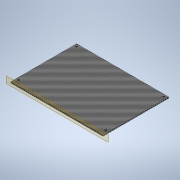
# Autodesk Inventor part: s_carbon_plate1
Saved by Autodesk Inventor 2022 (Build 260153000, 153)
## iProperties
Created: 2021-08-20
Part Number: s_carbon_plate1
Material: CFRP
Document SubType Name: Sheet Metal
Designer: yuta0
Density: 1.43 g/cm^3
Sheet Metal Rule: Default_mm
Appearance: カーボンファイバー
Mass: 103.386 g
Surface Area: 742.83 cm^2
Volume: 72.2979 cm^3
Author: yuta0
Autodesk Inventor part; units mm, degrees
ref_plane "YZ Plane" through (0, 0, 0) normal (1, 0, 0) x (0, 1, 0)
ref_plane "XZ Plane" through (0, 0, 0) normal (0, 1, 0) x (-1, 0, 0)
ref_plane "XY Plane" through (0, 0, 0) normal (0, 0, 1) x (1, 0, 0)
sketch "スケッチ1" plane through (0, 0, 0) normal (0, 1, 0) x (-1, 0, 0)
  line L0 (-87.5, 105) -> (87.5, 105)
  line L1 (87.5, 105) -> (87.5, -105)
  line L2 (87.5, -105) -> (-87.5, -105)
  line L3 (-87.5, -105) -> (-87.5, 105)
  line L4 (-87.5, 105) -> (87.5, -105) construction
  line L5 (87.5, 105) -> (-87.5, -105) construction
  point P0 (0, 0)
  dimension "d0" = 210
  dimension "d1" = 175
  measures "d0" distance of L0.end L1.end
  measures "d1" distance of L0.start L0.end
extrude "プレート1" add sketch "スケッチ1" along normal blind 2
sketch "スケッチ5" plane through (0, 2, 0) normal (0, 1, 0) x (1, 0, 0)
  line L0 (-24, -101) -> (34.6, -101)
  line L1 (34.6, -101) -> (34.6, -67)
  line L2 (34.6, -67) -> (-24, -67)
  line L3 (-24, -67) -> (-24, -101)
  line L4 (-24, -101) -> (34.6, -67) construction
  line L5 (34.6, -101) -> (-24, -67) construction
  line L6 (87.5, -105) -> (-87.5, -105) projected
  point P0 (0, 0)
  point P1 (0, -84)
  point P2 (5.3, -84)
  point P3 (5.3, -84)
  dimension "d31" = 58.6
  dimension "d32" = 24
  dimension "d33" = 34
  dimension "d78" = 4
  constraints: 12 end point, 3 midpoint, 2 parallel, 1 horizontal, 1 horizontal alignment, 1 perpendicular, 1 vertical alignment
  measures "d31" distance of L1.end L2.end
  measures "d32" distance from line of L3 point (0, -84)
  measures "d33" distance of L0.end L1.end
  measures "d78" distance between parallel lines of L6 L0
hole "穴3" at (34.6, 2, 67) at (34.6, 2, 101) at (-24, 2, 67) at (-24, 2, 101) direction (0, -1, 0) diameter 4.3 end through all clearance for "Socket Head Cap Screw" size "M4" standard "Ansi Metric M Profile"
sketch "スケッチ6" plane through (0, 2, 0) normal (0, 1, 0) x (1, 0, 0)
  line L0 (-133.9967, -217.2896) -> (133.2896, 49.9967)
  line L1 (133.2896, 49.9967) -> (133.9967, 49.2896)
  line L2 (133.9967, 49.2896) -> (-133.2896, -217.9967)
  line L3 (-133.2896, -217.9967) -> (-133.9967, -217.2896)
  line L4 (-133.9967, -217.2896) -> (133.9967, 49.2896) construction
  line L5 (133.2896, 49.9967) -> (-133.2896, -217.9967) construction
  line L6 (133.9967, -217.2896) -> (-133.2896, 49.9967)
  line L7 (-133.2896, 49.9967) -> (-133.9967, 49.2896)
  line L8 (-133.9967, 49.2896) -> (133.2896, -217.9967)
  line L9 (133.2896, -217.9967) -> (133.9967, -217.2896)
  line L10 (133.9967, -217.2896) -> (-133.9967, 49.2896) construction
  line L11 (-133.2896, 49.9967) -> (133.2896, -217.9967) construction
  line L12 (-2.4749, -82.2322) -> (-1.7678, -81.5251)
  circle A0 centre (0, -84) radius 22
  line L13 (2.4749, -82.2322) -> (1.7678, -81.5251)
  circle A1 centre (0, -84) radius 3
  line L14 (-87.5, -105) -> (-87.5, 105) projected
  line L15 (87.5, 105) -> (87.5, -105) projected
  line L16 (122.5, 0) -> (-122.5, 0) projected
  point P0 (0, 0)
  point P1 (0, -84)
  point P2 (-2.1213, -81.8787)
  point P3 (2.1213, -81.8787)
  point P4 (15.9059, -68.8012)
  point P5 (-15.9059, -68.8012)
  dimension "d54" = 1
  dimension "d55" = 1
  dimension "d57" = 44
  dimension "d59" = 3
  dimension "d60" = 3
  dimension "d65" = 186
  dimension "d66" = 186
  dimension "d79" = 45
  dimension "d80" = 45
  constraints: 28 end point, 5 midpoint, 4 parallel, 4 perpendicular, 4 point on line, 2 centre point, 2 coincident, 1 tangent
  measures "d54" distance between parallel lines of L6 L8
  measures "d55" distance between parallel lines of L0 L2
  measures "d57" diameter of A0
  measures "d59" distance from line of L12 A0.centre
  measures "d60" distance from line of L13 A0.centre
  measures "d65" distance between parallel lines of L7 L12
  measures "d66" distance between parallel lines of L1 L13
  measures "d79" angle of L6 L16
  measures "d80" angle of L16 L0
extrude "押し出し2" cut sketch "スケッチ6" against normal blind 10 contours A0 L6 L12 L8 | A0 L0 A1 L6 | L12 L6 A1 | A0 L2 L13 L0 | L0 L13 A1
sketch "スケッチ7" plane through (0, 2, 0) normal (0, 1, 0) x (1, 0, 0)
  line L0 (-82.5, -100) -> (82.5, -100)
  line L1 (82.5, -100) -> (82.5, 100)
  line L2 (82.5, 100) -> (-82.5, 100)
  line L3 (-82.5, 100) -> (-82.5, -100)
  line L4 (-82.5, -100) -> (82.5, 100) construction
  line L5 (82.5, -100) -> (-82.5, 100) construction
  line L6 (-87.5, -105) -> (-87.5, 105) projected
  line L7 (87.5, -105) -> (-87.5, -105) projected
  point P0 (0, 0)
  point P1 (-82.5, -45)
  point P2 (-82.5, -10)
  point P3 (82.5, -45)
  point P4 (82.5, -10)
  dimension "d45" = 5
  dimension "d46" = 5
  dimension "d67" = 55
  dimension "d68" = 35
  dimension "d69" = 55
  dimension "d70" = 35
  constraints: 12 end point, 4 point on line, 2 midpoint, 2 parallel, 1 horizontal, 1 perpendicular
  measures "d45" distance between parallel lines of L6 L3
  measures "d46" distance between parallel lines of L7 L0
  measures "d67" distance from line of L0 point (-82.5, -45)
  measures "d68" distance of point (-82.5, -10) point (-82.5, -45)
  measures "d69" distance from line of L0 point (82.5, -45)
  measures "d70" distance of point (82.5, -45) point (82.5, -10)
hole "穴4" at (-82.5, 2, -100) at (82.5, 2, -100) at (-82.5, 2, 100) at (82.5, 2, 100) direction (0, -1, 0) diameter 3.2 end through all clearance for "Socket Head Cap Screw" size "M3" standard "Ansi Metric M Profile"
sketch "スケッチ8" plane through (0, 2, 0) normal (0, 1, 0) x (1, 0, 0)
  line L0 (15.9059, -68.8012) -> (2.4749, -82.2322) projected
  line L1 (-2.1213, -81.8787) -> (-2.4749, -82.2322) projected
  arc A0 (2.1213, -81.8787) -> (-2.1213, -81.8787) centre (0, -84) ccw projected
  line L2 (2.4749, -82.2322) -> (2.1213, -81.8787) projected
  line L3 (-2.4749, -82.2322) -> (-15.9059, -68.8012) projected
  arc A1 (15.9059, -68.8012) -> (-15.9059, -68.8012) centre (0, -84) ccw projected
  line L4 (2.4749, -83.6464) -> (17.2895, -68.8318)
  arc A2 (17.2895, -68.8318) -> (-17.2895, -68.8318) centre (0, -84) ccw
  line L5 (-17.2895, -68.8318) -> (-2.4749, -83.6464)
  line L6 (-2.4749, -83.6464) -> (-1.4142, -82.5858)
  arc A3 (1.4142, -82.5858) -> (-1.4142, -82.5858) centre (0, -84) ccw
  line L7 (1.4142, -82.5858) -> (2.4749, -83.6464)
  point P0 (0, 0)
  dimension "d61" = 1
  constraints: 8 end point, 4 point on circle, 2 centre point, 5 other
  measures "d61" distance between parallel lines of L5 L3
extrude "押し出し3" cut sketch "スケッチ8" against normal blind 10 contours L0 L2 A0 L1 L3 A1 | L7 A3 L6 L5 A2 L4
fillet "コーナーR1" radius 1 4 edges at (-2.4749, 1, 83.6464) (2.4749, 1, 83.6464) (-17.2895, 1, 68.8318) (17.2895, 1, 68.8318)
hole "穴5" at (-82.5, 2, 45) at (-82.5, 2, 10) at (82.5, 2, 45) at (82.5, 2, 10) direction (0, -1, 0) diameter 3.4 end through all clearance for "Flat Head Machine Screw" size "M3" standard "Ansi Metric M Profile"
ref_plane "作業平面1" through (-87.5, 0, 20) normal (0, 0, 1) x (1, 0, 0)
sketch "スケッチ9" plane through (-87.5, 0, 20) normal (0, 0, 1) x (1, 0, 0)
  line L0 (175, 0) -> (175, 2) projected
  line L1 (0, 0) -> (175, 0)
  line L2 (175, 0) -> (175, 2)
  line L3 (175, 2) -> (0, 2)
  line L4 (0, 2) -> (0, 0)
  point P0 (87.5, 0)
  constraints: 8 end point, 2 parallel, 1 horizontal, 1 perpendicular
extrude "押し出し4" cut sketch "スケッチ9" along normal blind 159
equation "\"d40\" = Thickness"
equation "\"d60\" = d59"
equation "\"d66\" = d65"
equation "\"d69\" = d67"
equation "\"d70\" = d68"
equation "\"d76\" = Thickness"
equation "\"d2\" = Thickness"
equation "\"BendRadius\" = Thickness"
equation "\"BendReliefWidth\" = Thickness"
equation "\"BendReliefDepth\" = 0.5 * Thickness"
equation "\"CornerReliefSize\" = 4 * Thickness"
equation "\"MinimumRemnant\" = 2 * Thickness"
equation "\"TransitionRadius\" = BendRadius"
equation "\"JacobiRadiusSize\" = BendRadius"
equation "\"GapSize\" = Thickness"
equation "\"Thickness\" = 2"
